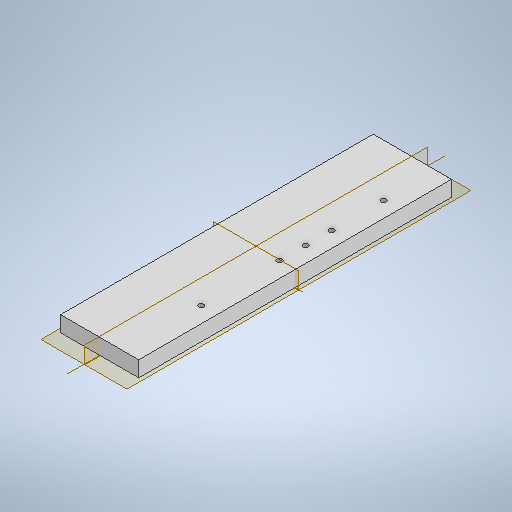
# Autodesk Inventor part: PrinterHeadLip_RightSide
Saved by Autodesk Inventor 2025 (Build 290162000, 162)
## iProperties
Created: 2024-06-06
Part Number: PrinterHeadLip_RightSide
Material: Generic
Document SubType Name: Modeling
Designer: mumin
Density: 1 g/cm^3
Appearance: Default
Author: mumin
Autodesk Inventor part; units mm, degrees
sketch "Sketch1" plane through (0, 0, 0) normal (0, 1, 0) x (-1, 0, 0)
  line L0 (37.5, 150) -> (-37.5, 150)
  line L1 (-37.5, 150) -> (-37.5, -150)
  line L2 (-37.5, -150) -> (37.5, -150)
  line L3 (37.5, -150) -> (37.5, 150)
  line L4 (37.5, 150) -> (-37.5, -150) construction
  line L5 (-37.5, 150) -> (37.5, -150) construction
  point P0 (0, 0)
  dimension "d0" = 75
  dimension "d1" = 300
  constraints: 12 end point, 2 midpoint, 2 parallel, 1 horizontal, 1 perpendicular
  measures "d0" distance of L2.end L1.end
  measures "d1" distance of L1.end L0.end
extrude "Extrusion1" add sketch "Sketch1" along normal blind 15
sketch "Sketch2" plane through (0, 15, 0) normal (0, 1, 0) x (1, 0, 0)
  line L0 (37.5, -150) -> (37.5, 150) projected
  line L1 (37.5, 150) -> (-37.5, 150) projected
  point P0 (0, 0)
  point P1 (22.5, 100)
  dimension "d11" = 15
  dimension "d12" = 50
  measures "d11" distance from line of L0 point (22.5, 100)
  measures "d12" distance from line of L1 point (22.5, 100)
hole "Hole1" at (22.5, 15, -100) direction (0, -1, 0) diameter 5 end through all
pattern_linear "Rectangular Pattern1" count 2 spacing 50 along (0, 0, 1) of "Hole1"
pattern_linear "Rectangular Pattern2" count 2 spacing 75 along (0, 0, 1) of "Hole1"
pattern_linear "Rectangular Pattern3" count 2 spacing 100 along (0, 0, 1) of "Hole1", "Rectangular Pattern2"
body "Solid1"
